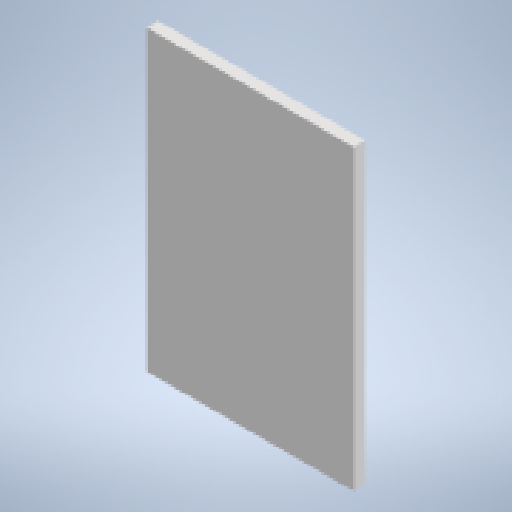
# Autodesk Inventor part: nan_holder
Saved by Autodesk Inventor 2024 (Build 280153000, 153)
## iProperties
Created: 2023-06-16
Part Number: nan_holder
Material: Generic
Document SubType Name: Modeling
Designer: Rober
Density: 1 g/cm^3
Appearance: Default
Author: Rober
Autodesk Inventor part; units mm, degrees
ref_plane "YZ Plane" through (0, 0, 0) normal (1, 0, 0) x (0, 1, 0)
ref_plane "XZ Plane" through (0, 0, 0) normal (0, 1, 0) x (-1, 0, 0)
ref_plane "XY Plane" through (0, 0, 0) normal (0, 0, 1) x (1, 0, 0)
sketch "Sketch1" plane through (0, 0, 0) normal (0, 0, 1) x (1, 0, 0)
  line L0 (8.8842, 16.4234) -> (-8.8842, 16.4234)
  line L1 (-8.8842, 16.4234) -> (-8.8842, 41.9995)
  line L2 (-8.8842, 41.9995) -> (8.8842, 41.9995)
  line L3 (8.8842, 41.9995) -> (8.8842, 16.4234)
  arc A0 (5.5604, 35.6068) -> (5.5604, 37.8906) centre (5.5604, 36.7487) ccw projected
  line L4 (-5.5604, 35.6068) -> (5.5604, 35.6068) projected
  arc A1 (-5.5604, 37.8906) -> (-5.5604, 35.6068) centre (-5.5604, 36.7487) ccw projected
  line L5 (5.5604, 37.8906) -> (-5.5604, 37.8906) projected
  line L6 (5.5604, -35.6068) -> (-5.5604, -35.6068) projected
  arc A2 (5.5604, -37.8906) -> (5.5604, -35.6068) centre (5.5604, -36.7487) ccw projected
  line L7 (-5.5604, -37.8906) -> (5.5604, -37.8906) projected
  arc A3 (-5.5604, -35.6068) -> (-5.5604, -37.8906) centre (-5.5604, -36.7487) ccw projected
  arc A4 (-8.8842, 18.7594) -> (-15.14, 6.5) centre (0, 6.5) ccw projected
  line L8 (-15.14, -6.5) -> (-15.14, 6.5) projected
  arc A5 (-15.14, -6.5) -> (-8.8842, -18.7594) centre (0, -6.5) ccw projected
  line L9 (-8.8842, -40.7487) -> (-8.8842, -18.7594) projected
  line L10 (8.8842, -40.7487) -> (-8.8842, -40.7487) projected
  line L11 (8.8842, -18.7594) -> (8.8842, -40.7487) projected
  arc A6 (8.8842, -18.7594) -> (15.14, -6.5) centre (0, -6.5) ccw projected
  line L12 (15.14, 6.5) -> (15.14, -6.5) projected
  arc A7 (15.14, 6.5) -> (8.8842, 18.7594) centre (0, 6.5) ccw projected
  line L13 (8.8842, 40.7487) -> (8.8842, 18.7594) projected
  line L14 (-8.8842, 40.7487) -> (8.8842, 40.7487) projected
  line L15 (-8.8842, 18.7594) -> (-8.8842, 40.7487) projected
  arc A8 (-12, -6.5) -> (12, -6.5) centre (0, -6.5) ccw projected
  line L16 (-12, 6.5) -> (-12, -6.5) projected
  arc A9 (12, 6.5) -> (-12, 6.5) centre (0, 6.5) ccw projected
  line L17 (12, -6.5) -> (12, 6.5) projected
  point P0 (0, 0)
  point P1 (8.8842, 29.2114)
  constraints: 8 end point, 4 parallel, 1 horizontal, 1 midpoint, 1 perpendicular, 1 point on line
extrude "Extrusion1" add sketch "Sketch1" along normal blind 1 contours L0 A9 L1 L14 L3 | L0 A9 | L14 L1 L2 L3 | L4 A1 L5 A0
body "Solid1"
